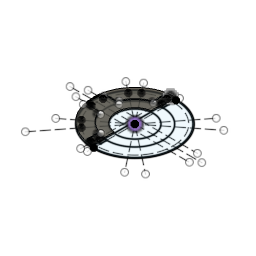
sphere2_base v7 (Autodesk Fusion 360 design; units mm, degrees)
Autodesk Fusion 360 part; units mm, degrees
sketch "Skizze1" plane through (0, 0, 0) normal (0, 0, 1) x (1, 0, 0)
  circle A0 centre (0, 0) radius 71.5
  line L0 (-110.8063, 0) -> (114.3399, 0) construction
  line L1 (0, 76.1004) -> (0, -81.1485) construction
  line L2 (-68, 15.2) -> (-42.2202, 15.2)
  line L3 (-73, -15.2) -> (-43.4634, -15.2)
  line L4 (-15.2, -68.5347) -> (-15.2, -43)
  line L5 (-15.2, 68) -> (-15.2, 46.5327)
  line L6 (-4, 71.388) -> (-4, -71.388)
  circle A1 centre (0, 0) radius 65 construction
  line L7 (-10, -82.6476) -> (-10, 70.8393) construction
  line L8 (-90, 10) -> (96.6694, 10) construction
  line L9 (-90.7656, -10) -> (103.0696, -10) construction
  circle A2 centre (-10, -64.2262) radius 1.75
  circle A3 centre (-64.2262, -10) radius 1.75
  circle A4 centre (-64.2262, 10) radius 1.75
  circle A5 centre (-10, 64.2262) radius 1.75
  line L10 (-75.8849, -59.2878) -> (85.2533, 66.6071) construction
  circle A6 centre (-51.2207, -40.018) radius 1.75
  circle A7 centre (0, 0) radius 48
  circle A8 centre (0, 0) radius 70.2
  circle A9 centre (-18.2, -47.642) radius 3
  circle A10 centre (-47.642, -18.2) radius 3
  circle A11 centre (-66.0833, 12.2) radius 3
  circle A12 centre (-47.642, 18.2) radius 3
  circle A13 centre (-66.0833, -12.2) radius 3
  circle A14 centre (-12.2, -66.0833) radius 3
  circle A15 centre (-18.2, 47.642) radius 3
  circle A16 centre (-12.2, 66.0833) radius 3
  circle A17 centre (0, 0) radius 31.5
  line L11 (-8, 58.2) -> (0, 58.2)
  line L12 (0, 58.2) -> (0, 48.2)
  line L13 (0, 48.2) -> (-8, 48.2)
  line L14 (-10, 50.2) -> (-10, 56.2)
  arc A18 (-8, 58.2) -> (-10, 56.2) centre (-8, 56.2) ccw
  arc A19 (-10, 50.2) -> (-8, 48.2) centre (-8, 50.2) ccw
  line L15 (-8, -48.2) -> (0, -48.2)
  line L16 (0, -48.2) -> (0, -58.2)
  line L17 (0, -58.2) -> (-8, -58.2)
  line L18 (-10, -56.2) -> (-10, -50.2)
  arc A20 (-8, -48.2) -> (-10, -50.2) centre (-8, -50.2) ccw
  arc A21 (-10, -56.2) -> (-8, -58.2) centre (-8, -56.2) ccw
  line L19 (-82.0813, -105.0592) -> (60.9272, 77.9833) construction
  circle A22 centre (-40.018, -51.2207) radius 1.75
  line L20 (-53.2096, 68.1052) -> (62.591, -80.1128) construction
  line L21 (-70.5143, 55.0918) -> (83.1243, -64.9438) construction
  circle A23 centre (-40.018, 51.2207) radius 1.75
  circle A24 centre (-51.2207, 40.018) radius 1.75
  point P0 (-10, -64.2262)
  point P1 (-10, 70.8393)
  point P2 (-10, 64.2262)
  point P3 (-64.2262, 10)
  point P4 (-64.2262, -10)
  point P5 (-51.2207, -40.018)
  point P6 (-47.5633, 20.7568)
  point P7 (0, 70.2)
  point P8 (0, -70.2)
  point P9 (-40.018, -51.2207)
  point P10 (-51.2207, 40.018)
  point P11 (-40.018, 51.2207)
  dimension "d1" = 143
  dimension "d4" = 15.2
  dimension "d8" = 15.2
  dimension "d9" = 15.2
  dimension "d10" = 15.2
  dimension "d28" = 4
  dimension "d30" = 130
  dimension "d32" = 10
  dimension "d33" = 10
  dimension "d34" = 10
  dimension "d35" = 3.5
  dimension "d40" = 3.5
  dimension "d41" = 3.5
  dimension "d42" = 3.5
  dimension "d53" = 38
  dimension "d58" = 3.5
  dimension "d67" = 96
  dimension "d81" = 140.4
  dimension "d82" = 6
  dimension "d83" = 6
  dimension "d85" = 6
  dimension "d87" = 6
  dimension "d88" = 6
  dimension "d89" = 6
  dimension "d90" = 6
  dimension "d91" = 6
  dimension "d92" = 63
  dimension "d93" = 12
  dimension "d94" = 10
  dimension "d95" = 10
  dimension "d96" = 2
  dimension "d97" = 12
  dimension "d98" = 10
  dimension "d99" = 10
  dimension "d100" = 2
  dimension "d109" = 38
  dimension "d110" = 3.5
  dimension "d111" = 15.843
  dimension "d115" = 38
  dimension "d116" = 38
  dimension "d117" = 3.5
  dimension "d118" = 3.5
  dimension "d119" = 15.843
  constraint coincident A0.centre A1.centre
  constraint horizontal L0
  constraint vertical L1
  constraint coincident A0.centre L1
  constraint perpendicular L1 L2
  constraint horizontal L3
  constraint vertical L4
  constraint vertical L5
  constraint vertical L6
  constraint coincident A0 L6.start
  constraint coincident A0 L6.end
  constraint vertical L7
  constraint coincident A1 P0
  constraint coincident L7 P0
  constraint coincident P1 L7.end
  constraint coincident L7 P2
  constraint coincident A1 P2
  constraint horizontal L8
  constraint horizontal L9
  constraint coincident A1 P3
  constraint coincident L8 P3
  constraint coincident A1 P4
  constraint coincident L9 P4
  constraint coincident P0 A2.centre
  constraint coincident P4 A3.centre
  constraint coincident P3 A4.centre
  constraint coincident P2 A5.centre
  constraint coincident L10 P5
  constraint coincident A1 P5
  constraint coincident P5 A6.centre
  constraint tangent A7 A9
  constraint tangent L4 A9
  constraint tangent L3 A10
  constraint tangent A7 A10
  constraint tangent L2 A11
  constraint tangent A8 A11
  constraint tangent L2 A12
  constraint tangent A7 A12
  constraint tangent L3 A13
  constraint tangent A8 A13
  constraint coincident L4.start A8
  constraint tangent A8 A14
  constraint tangent L4 A14
  constraint tangent A7 A15
  constraint tangent L5 A15
  constraint tangent L5 A16
  constraint tangent A8 A16
  constraint concentric A8 A17
  constraint horizontal L11
  constraint vertical L12
  constraint horizontal L13
  constraint vertical L14
  constraint coincident A8 P7
  constraint coincident L1 P7
  constraint coincident L1 L11.end
  constraint tangent L11 A18
  constraint tangent L14 A18
  constraint tangent L13 A19
  constraint tangent L14 A19
  constraint equal A18 A19
  constraint horizontal L15
  constraint vertical L16
  constraint horizontal L17
  constraint vertical L18
  constraint coincident A8 P8
  constraint coincident L1 P8
  constraint coincident L1 L16.end
  constraint tangent L15 A20
  constraint tangent L18 A20
  constraint tangent L17 A21
  constraint tangent L18 A21
  constraint equal A20 A21
  constraint coincident L0 A0.centre
  constraint coincident A0.centre L10
  constraint coincident A0.centre L19
  constraint coincident L19 P9
  constraint coincident A1 P9
  constraint coincident P9 A22.centre
  constraint coincident A0.centre L20
  constraint coincident A0.centre L21
  constraint coincident A1 P10
  constraint coincident A1 P11
  constraint coincident L20 P11
  constraint coincident L21 P10
  constraint coincident P11 A23.centre
  constraint coincident P10 A24.centre
  measures "d1" diameter of A0
  measures "d4" distance of L1 L5
  measures "d8" distance of L1 L4
  measures "d9" distance of L0 L3
  measures "d10" distance of L0 L2
  measures "d28" distance of L1 L6
  measures "d30" diameter of A1
  measures "d32" distance of L1 L7
  measures "d33" distance of L0 L9
  measures "d34" distance of L0 L8
  measures "d35" diameter of A5
  measures "d40" diameter of A2
  measures "d41" diameter of A3
  measures "d42" diameter of A4
  measures "d53" angle of L0 L10
  measures "d58" diameter of A6
  measures "d67" diameter of A7
  measures "d81" diameter of A8
  measures "d82" diameter of A9
  measures "d83" diameter of A10
  measures "d85" diameter of A11
  measures "d87" diameter of A12
  measures "d88" diameter of A13
  measures "d89" diameter of A14
  measures "d90" diameter of A15
  measures "d91" diameter of A16
  measures "d92" diameter of A17
  measures "d93" distance of L11 P7
  measures "d94" distance of L11 L13
  measures "d95" distance of L12 L14
  measures "d96" radius of A18
  measures "d97" distance of L17 P8
  measures "d98" distance of L15 L17
  measures "d99" distance of L16 L18
  measures "d100" radius of A20
  measures "d109" angle of L1 L19
  measures "d110" diameter of A22
  measures "d111" distance of P5 P9
  measures "d115" angle of L1 L20
  measures "d116" angle of L0 L21
  measures "d117" diameter of A24
  measures "d118" diameter of A23
  measures "d119" distance of P11 P10
extrude "Extrusion3" add sketch "Skizze1" along normal blind 2 contours L5 L6 A5 A7 A8 A15 A16 L11 L13 L14 A18 A19 | L4 L6 A2 A7 A8 A14 L15 L17 L18 A20 A21 | A5 A16 | A2 A14 | L2 L3 A3 A4 A7 A8 A11 A13 | A3 A13 | A4 A11 | L3 A7 A10 | L6 A7 A17 | L4 A7 A9 | L2 A7 A12 picked at (-12.0699, 67.885) picked at (-12.0699, -67.885) picked at (-67.2201, -13.3537) picked at (-67.2201, 13.3537) picked at (-38.4795, 17.8579)
extrude "Extrusion4" add sketch "Skizze1" along normal blind 3.6 contours A0 L3 L6 A8 | A0 L3 L6 A8 | L3 A8 A13 | L3 L4 A7 A8 A9 A10 | L2 L5 A7 A8 A11 A12 A15 A16 | L4 A8 A14 | A10 | A15 | A9 | A12
